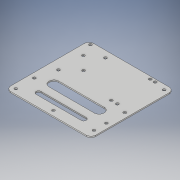
# Autodesk Inventor part: Tier4
Saved by Autodesk Inventor 2018 (Build 220112000, 112)
## iProperties
Created: 2019-03-27
Part Number: Tier4
Material: Generic
Document SubType Name: Modeling
Designer: anirudh
Density: 1 g/cm^3
Appearance: Default
Author: anirudh
Autodesk Inventor part; units mm, degrees
ref_plane "YZ Plane" through (0, 0, 0) normal (1, 0, 0) x (0, 1, 0)
ref_plane "XZ Plane" through (0, 0, 0) normal (0, 1, 0) x (-1, 0, 0)
ref_plane "XY Plane" through (0, 0, 0) normal (0, 0, 1) x (1, 0, 0)
sketch "Sketch1" plane through (0, 0, 0) normal (0, 1, 0) x (-1, 0, 0)
  line L0 (0, 0) -> (108.585, 0)
  line L1 (108.585, 0) -> (108.585, -106.045)
  line L2 (108.585, -106.045) -> (0, -106.045)
  line L3 (0, -106.045) -> (0, 0)
  dimension "d0" = 108.585
  dimension "d1" = 106.045
  constraints: 8 end point, 2 parallel, 1 horizontal, 1 perpendicular
  measures "d0" distance of L1.end L2.end
  measures "d1" distance of L0.end L1.end
extrude "Extrusion1" add sketch "Sketch1" along normal blind 1.5875
fillet "Fillet1" radius 6.35 4 edges at (0, 0.7937, 0) (0, 0.7937, -106.045) (-108.585, 0.7937, -106.045) (-108.585, 0.7937, 0)
sketch "Sketch2" plane through (0, 1.5875, 0) normal (0, 1, 0) x (1, 0, 0)
  line L0 (0, 6.35) -> (0, 99.695) projected
  circle A0 centre (-20.6756, 102.616) radius 1.8
  circle A1 centre (-20.6756, 54.2798) radius 1.8
  circle A2 centre (-95.8088, 54.2798) radius 1.8
  circle A3 centre (-103.3018, 102.616) radius 1.8
  point P0 (0, 0)
  dimension "d8" = 3.6
  dimension "d10" = 3.6
  dimension "d12" = 3.6
  dimension "d14" = 3.6
  constraints: 4 centre point
  measures "d8" diameter of A0
  measures "d10" diameter of A1
  measures "d12" diameter of A2
  measures "d14" diameter of A3
extrude "Extrusion2" cut sketch "Sketch2" against normal blind 1.5875
sketch "Sketch5" plane through (0, 1.5875, 0) normal (0, 1, 0) x (1, 0, 0)
  arc A0 (-108.585, 6.35) -> (-102.235, 0) centre (-102.235, 6.35) ccw projected
  circle A1 centre (-102.235, 6.35) radius 1.8
  circle A2 centre (-6.35, 6.35) radius 1.8 projected
  circle A3 centre (-6.35, 45.72) radius 1.8 projected
  circle A4 centre (-54.2925, 6.35) radius 1.8
  circle A5 centre (-6.35, 26.035) radius 1.8
  arc A6 (0, 99.695) -> (-6.35, 106.045) centre (-6.35, 99.695) ccw projected
  circle A7 centre (-6.35, 99.695) radius 1.8
  circle A8 centre (-95.8088, 54.2798) radius 1.8 projected
  circle A9 centre (-95.8088, 86.0298) radius 1.8
  point P0 (0, 0)
  dimension "d23" = 3.6
  dimension "d24" = 3.6
  dimension "d25" = 3.6
  dimension "d26" = 3.6
  dimension "d28" = 3.6
  constraints: 5 centre point, 2 coincident
  measures "d23" diameter of A1
  measures "d24" diameter of A4
  measures "d25" diameter of A5
  measures "d26" diameter of A7
  measures "d28" diameter of A9
extrude "Extrusion4" cut sketch "Sketch5" against normal blind 1.5875 contours A1 | A4 | A5 | A7 | A9
sketch "Sketch6" plane through (0, 1.5875, 0) normal (0, 1, 0) x (1, 0, 0)
  circle A0 centre (-6.35, 6.35) radius 1.8 projected
  circle A1 centre (-6.35, 26.035) radius 1.8 projected
  circle A2 centre (-102.235, 6.35) radius 1.8 projected
  circle A3 centre (-102.235, 26.035) radius 1.8 projected
  arc A4 (-83.185, 19.3675) -> (-83.185, 13.0175) centre (-83.185, 16.1925) ccw
  arc A5 (-25.4, 13.0175) -> (-25.4, 19.3675) centre (-25.4, 16.1925) ccw
  line L0 (-25.4, 19.3675) -> (-83.185, 19.3675)
  line L1 (-83.185, 13.0175) -> (-25.4, 13.0175)
  circle A6 centre (-6.35, 45.72) radius 1.8 projected
  arc A7 (-83.185, 42.2275) -> (-83.185, 29.5275) centre (-83.185, 35.8775) ccw
  arc A8 (-25.4, 29.5275) -> (-25.4, 42.2275) centre (-25.4, 35.8775) ccw
  line L2 (-83.185, 29.5275) -> (-25.4, 29.5275)
  line L3 (-25.4, 42.2275) -> (-83.185, 42.2275)
  point P0 (0, 0)
  dimension "d33" = 6.35
  dimension "d34" = 6.35
  dimension "d37" = 12.7
  dimension "d38" = 12.7
  constraints: 8 end point, 8 point on circle, 4 centre point, 2 horizontal, 2 parallel
  measures "d33" diameter of A4
  measures "d34" diameter of A5
  measures "d37" diameter of A7
  measures "d38" diameter of A8
extrude "Extrusion5" cut sketch "Sketch6" against normal blind 1.5875 contours L0 A5 L1 A4 | L3 A8 L2 A7
sketch "Sketch7" plane through (0, 1.5875, 0) normal (0, 1, 0) x (1, 0, 0)
  circle A0 centre (-27.0256, 102.616) radius 1.8
  circle A1 centre (-28.4226, 54.2798) radius 1.8
  point P0 (0, 0)
  dimension "d42" = 3.6
  dimension "d46" = 3.6
  constraints: 2 centre point
  measures "d42" diameter of A0
  measures "d46" diameter of A1
extrude "Extrusion6" cut sketch "Sketch7" against normal blind 25.4
sketch "Sketch8" plane through (0, 1.5875, 0) normal (0, 1, 0) x (1, 0, 0)
  line L0 (-108.585, 99.695) -> (-108.585, 6.35) projected
  line L1 (-102.235, 106.045) -> (-6.35, 106.045) projected
  circle A0 centre (-79.0956, 97.536) radius 1.8
  circle A1 centre (-79.0956, 69.596) radius 1.8
  point P0 (0, 0)
  dimension "d51" = 3.6
  dimension "d53" = 3.6
  constraints: 2 centre point
  measures "d51" diameter of A0
  measures "d53" diameter of A1
extrude "Extrusion7" cut sketch "Sketch8" against normal blind 25.4
sketch "Sketch10" plane through (0, 1.5875, 0) normal (0, 1, 0) x (1, 0, 0)
  circle A0 centre (-6.35, 12.7) radius 1.8 projected
  circle A1 centre (-6.35, 52.07) radius 1.8 projected
  circle A2 centre (-102.235, 32.385) radius 1.8 projected
  circle A3 centre (-102.235, 29.845) radius 1.8
  circle A4 centre (-6.35, 10.16) radius 1.8
  circle A5 centre (-6.35, 49.53) radius 1.8
  point P0 (0, 0)
  dimension "d67" = 3.6
  dimension "d68" = 3.6
  dimension "d69" = 3.6
  constraints: 3 centre point
  measures "d67" diameter of A3
  measures "d68" diameter of A4
  measures "d69" diameter of A5
extrude "Extrusion9" cut sketch "Sketch10" against normal blind 25.4 contours A4 A0 | A0 A4 | A5 A1 | A1 A5 | A3 A2 | A2 A3 picked at (-6.4174, 11.6029) picked at (-6.4455, 9.2198) picked at (-6.4174, 50.9729) picked at (-6.4455, 48.5898) picked at (-102.3024, 31.2879) picked at (-102.3305, 28.9048)
sketch "Sketch11" plane through (0, 1.5875, 0) normal (0, 1, 0) x (1, 0, 0)
  arc A0 (-6.35, 0) -> (0, 6.35) centre (-6.35, 6.35) ccw projected
  arc A1 (-108.585, 6.35) -> (-102.235, 0) centre (-102.235, 6.35) ccw projected
  arc A2 (-108.585, 6.35) -> (-102.235, 0) centre (-102.235, 6.35) ccw
  circle A3 centre (-102.235, 6.35) radius 1.8
  circle A4 centre (-102.235, 29.845) radius 1.8 projected
  circle A5 centre (-102.235, 29.845) radius 1.8
  circle A6 centre (-95.8088, 54.2798) radius 1.8 projected
  circle A7 centre (-95.8088, 54.2798) radius 1.8
  circle A8 centre (-95.8088, 86.0298) radius 1.8 projected
  circle A9 centre (-95.8088, 86.0298) radius 1.8
  circle A10 centre (-103.3018, 102.616) radius 1.8 projected
  circle A11 centre (-103.3018, 102.616) radius 1.8
  arc A12 (-102.235, 106.045) -> (-108.585, 99.695) centre (-102.235, 99.695) ccw projected
  arc A13 (-102.235, 106.045) -> (-108.585, 99.695) centre (-102.235, 99.695) ccw
  circle A14 centre (-20.6756, 54.2798) radius 1.8 projected
  circle A15 centre (-20.6756, 54.2798) radius 1.8
  circle A16 centre (-79.0956, 69.596) radius 1.8 projected
  circle A17 centre (-79.0956, 69.596) radius 1.8
  circle A18 centre (-79.0956, 97.536) radius 1.8 projected
  circle A19 centre (-79.0956, 97.536) radius 1.8
  circle A20 centre (-28.4226, 54.2798) radius 1.8 projected
  circle A21 centre (-28.4226, 54.2798) radius 1.8
  circle A22 centre (-27.0256, 102.616) radius 1.8 projected
  circle A23 centre (-27.0256, 102.616) radius 1.8
  circle A24 centre (-20.6756, 102.616) radius 1.8 projected
  circle A25 centre (-20.6756, 102.616) radius 1.8
  circle A26 centre (-6.35, 99.695) radius 1.8 projected
  circle A27 centre (-6.35, 99.695) radius 1.8
  arc A28 (0, 99.695) -> (-6.35, 106.045) centre (-6.35, 99.695) ccw projected
  arc A29 (0, 99.695) -> (-6.35, 106.045) centre (-6.35, 99.695) ccw
  arc A30 (-6.35, 0) -> (0, 6.35) centre (-6.35, 6.35) ccw
  circle A31 centre (-6.35, 10.16) radius 1.8 projected
  circle A32 centre (-6.35, 10.16) radius 1.8
  circle A33 centre (-6.35, 26.035) radius 1.8 projected
  circle A34 centre (-6.35, 26.035) radius 1.8
  circle A35 centre (-6.35, 49.53) radius 1.8 projected
  circle A36 centre (-6.35, 49.53) radius 1.8
  circle A37 centre (-54.2925, 6.35) radius 1.8 projected
  circle A38 centre (-54.2925, 6.35) radius 1.8
  line L0 (-6.35, 0) -> (-102.235, 0) projected
  line L1 (-6.35, 0) -> (-102.235, 0)
  line L2 (-108.585, 6.35) -> (-108.585, 99.695) projected
  line L3 (-108.585, 6.35) -> (-108.585, 99.695)
  line L4 (-102.235, 106.045) -> (-6.35, 106.045) projected
  line L5 (-102.235, 106.045) -> (-6.35, 106.045)
  line L6 (0, 99.695) -> (0, 6.35) projected
  line L7 (0, 99.695) -> (0, 6.35)
  point P0 (0, 0)
  constraints: 20 centre point, 20 coincident, 8 end point, 8 point on circle, 6 tangent, 3 collinear, 1 horizontal
body "Solid1"
